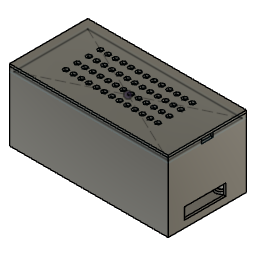
Raspberry Pi Zero W Case v16 (Autodesk Fusion 360 design; units mm, degrees)
Autodesk Fusion 360 part; units mm, degrees
note: some values were not read from the file. Chosen so that the rebuilt part matches the saved one: which face or edge a step refers to.
box "BoxPrimitive1" add length 34 width 69 height 30 placed x (0, -1, 0) y (1, 0, 0) z (0, 0, 1) at (-30, 15, 0) makes body 1
move_body "Align2" bodies 1 to x (1, 0, 0) y (0, 1, 0) z (0, 0, 1) at (-4.5, 2, 0)
shell "Shell1" thickness 1 removed faces 1 at (11.5, 5.6667, 30) on bodies 1
sketch "Sketch2" plane through (0, 0, 1) normal (0, 0, 1) x (-1, 0, 0)
  line L0 (33.5, 16) -> (-33.5, 16)
  line L1 (-33.5, 16) -> (-33.5, -16)
  line L2 (-33.5, -16) -> (33.5, -16)
  line L3 (33.5, -16) -> (33.5, 16)
  circle A0 centre (29, -11.5) radius 2.5
  circle A1 centre (29, -11.5) radius 1.25
  circle A2 through (29.5, -11.5, 4) (28.75, -11.067, 4) (28.75, -11.933, 4)
  dimension "d7" = 5
  dimension "d8" = 4.5
  dimension "d9" = 4.5
  dimension "d10" = 2.5
  dimension "d11" = 1
  constraint concentric A0 A1
  measures "d7" diameter of A0
  measures "d8" distance of L2 A0.centre
  measures "d9" distance of L3 A0.centre
  measures "d10" diameter of A1
sketch "Sketch2 (curves 4 mm off its plane)" plane through (0, 0, 5) normal (0, 0, 1) x (-1, 0, 0)
  circle A0 centre (29, -11.5) radius 0.5
loft "Loft1" add profiles "Sketch2", "Sketch2 (curves 4 mm off its plane)" section 1 contours A1 section 2 bodies 1
extrude "Extrude1" add sketch "Sketch2" along normal blind 1 contours A0 bodies 1
pattern_linear "R-Pattern1" count 2 spacing 58 along (1, 0, 0) count 2 spacing 23 along (0, -1, 0) of 4 faces at (-28.2726, 12.4121, 1.4444) (-29.287, 11.6721, 5) (-31.0694, 11.6863, 2) (-31.4876, 11.7489, 1.6667) on bodies 1
sketch "Sketch3" plane through (0, 17, 0) normal (0, 1, 0) x (-1, 0, 0)
  line L0 (-34.5, 30) -> (-34.5, 0)
  line L1 (-34.5, 0) -> (34.5, 0)
  line L2 (34.5, 0) -> (34.5, 30)
  line L3 (34.5, 30) -> (-34.5, 30)
  line L4 (-13.6, 8) -> (-28.6, 8)
  line L5 (-28.6, 8) -> (-28.6, 3)
  line L6 (-28.6, 3) -> (-13.6, 3)
  line L7 (-13.6, 3) -> (-13.6, 8)
  line L8 (-13.6, 8) -> (-28.6, 3) construction
  line L9 (-28.6, 8) -> (-13.6, 3) construction
  line L10 (2.9, 8) -> (12.9, 8)
  line L11 (12.9, 8) -> (12.9, 3)
  line L12 (12.9, 3) -> (2.9, 3)
  line L13 (2.9, 3) -> (2.9, 8)
  line L14 (2.9, 8) -> (12.9, 3) construction
  line L15 (12.9, 8) -> (2.9, 3) construction
  line L16 (25.5, 3) -> (15.5, 3)
  line L17 (15.5, 3) -> (15.5, 8)
  line L18 (15.5, 8) -> (25.5, 8)
  line L19 (25.5, 8) -> (25.5, 3)
  line L20 (25.5, 3) -> (15.5, 8) construction
  line L21 (15.5, 3) -> (25.5, 8) construction
  point P0 (-21.1, 5.5)
  point P1 (7.9, 5.5)
  point P2 (20.5, 5.5)
  dimension "d18" = 15
  dimension "d19" = 5
  dimension "d20" = 13.4
  dimension "d21" = 5.5
  dimension "d22" = 10
  dimension "d23" = 5
  dimension "d24" = 42.4
  dimension "d25" = 5.5
  dimension "d26" = 10
  dimension "d27" = 5
  dimension "d28" = 5.5
  dimension "d29" = 55
  constraint horizontal L4
  constraint perpendicular L4 L5
  constraint parallel L4 L6
  constraint parallel L5 L7
  constraint coincident L8 P0
  constraint coincident L9 P0
  constraint horizontal L10
  constraint perpendicular L10 L11
  constraint parallel L10 L12
  constraint parallel L11 L13
  constraint coincident L14 P1
  constraint coincident L15 P1
  constraint horizontal L16
  constraint perpendicular L16 L17
  constraint parallel L16 L18
  constraint parallel L17 L19
  constraint coincident L20 P2
  constraint coincident L21 P2
  measures "d18" distance of L5.end L6.end
  measures "d19" distance of L4.end L5.end
  measures "d20" distance of L0 P0
  measures "d21" distance of L1 P0
  measures "d22" distance of L11.end L12.end
  measures "d23" distance of L10.end L11.end
  measures "d24" distance of L0 P1
  measures "d25" distance of L1 P1
  measures "d26" distance of L17.end L18.end
  measures "d27" distance of L16.end L17.end
  measures "d28" distance of L1 P2
  measures "d29" distance of L0 P2
sketch "Sketch4" plane through (34.5, 0, 0) normal (1, 0, 0) x (0, 1, 0)
  line L0 (-17, 30) -> (-17, 0)
  line L1 (-17, 0) -> (17, 0)
  line L2 (17, 0) -> (17, 30)
  line L3 (17, 30) -> (-17, 30)
  line L4 (8.1, 8) -> (-9.9, 8)
  line L5 (-9.9, 8) -> (-9.9, 3)
  line L6 (-9.9, 3) -> (8.1, 3)
  line L7 (8.1, 3) -> (8.1, 8)
  line L8 (8.1, 8) -> (-9.9, 3) construction
  line L9 (-9.9, 8) -> (8.1, 3) construction
  line L10 (17, 30) -> (17, 0)
  point P0 (-0.9, 5.5)
  dimension "d30" = 18
  dimension "d31" = 5
  dimension "d32" = 17.9
  dimension "d33" = 5.5
  constraint horizontal L4
  constraint perpendicular L4 L5
  constraint parallel L4 L6
  constraint parallel L5 L7
  constraint coincident L8 P0
  constraint coincident L9 P0
  measures "d30" distance of L5.end L6.end
  measures "d31" distance of L4.end L5.end
  measures "d32" distance of P0 L10
  measures "d33" distance of L1 P0
extrude "Extrude2" cut sketch "Sketch3" against normal blind 1 contours L4 L5 L6 L7 | L10 L11 L12 L13 | L16 L17 L18 L19 bodies 1
extrude "Extrude3" cut sketch "Sketch4" against normal blind 1 contours L4 L5 L6 L7 bodies 1
sketch "Sketch5" plane through (34.5, 0, 0) normal (1, 0, 0) x (0, 1, 0)
  line L0 (-9.9, 8) -> (8.1, 8)
  line L1 (8.1, 8) -> (8.1, 3)
  line L2 (8.1, 3) -> (-9.9, 3)
  line L3 (-9.9, 3) -> (-9.9, 8)
  line L4 (-17, 30) -> (-17, 0)
  line L5 (-17, 0) -> (17, 0)
  line L6 (17, 0) -> (17, 30)
  line L7 (17, 30) -> (-17, 30)
  line L8 (2.5, 30) -> (-2.5, 30)
  line L9 (-2.5, 30) -> (-2.5, 28)
  line L10 (-2.5, 28) -> (2.5, 28)
  line L11 (2.5, 28) -> (2.5, 30)
  line L12 (2.5, 30) -> (-2.5, 28) construction
  line L13 (-2.5, 30) -> (2.5, 28) construction
  point P0 (0, 29)
  dimension "d38" = 5
  dimension "d39" = 2
  dimension "d40" = 17
  dimension "d41" = 1
  constraint horizontal L8
  constraint perpendicular L8 L9
  constraint parallel L8 L10
  constraint parallel L9 L11
  constraint coincident L12 P0
  constraint coincident L13 P0
  measures "d38" distance of L9.end L10.end
  measures "d39" distance of L8.end L9.end
  measures "d40" distance of L4 P0
  measures "d41" distance of L7 P0
extrude "Extrude4" cut sketch "Sketch5" against normal blind 1 contours L7 L8 L9 L10 L11 bodies 1
sketch "Sketch6" plane through (-34.5, 0, 0) normal (-1, 0, 0) x (0, -1, 0)
  line L0 (-17, 30) -> (-17, 0)
  line L1 (-17, 0) -> (17, 0)
  line L2 (17, 0) -> (17, 30)
  line L3 (17, 30) -> (-17, 30)
  line L4 (2.5, 28) -> (-2.5, 28)
  line L5 (-2.5, 28) -> (-2.5, 30)
  line L6 (-2.5, 30) -> (2.5, 30)
  line L7 (2.5, 30) -> (2.5, 28)
  line L8 (2.5, 28) -> (-2.5, 30) construction
  line L9 (-2.5, 28) -> (2.5, 30) construction
  point P0 (0, 29)
  dimension "d44" = 5
  dimension "d45" = 2
  dimension "d46" = 17
  dimension "d47" = 1
  constraint horizontal L4
  constraint perpendicular L4 L5
  constraint parallel L4 L6
  constraint parallel L5 L7
  constraint coincident L8 P0
  constraint coincident L9 P0
  measures "d44" distance of L5.end L6.end
  measures "d45" distance of L4.end L5.end
  measures "d46" distance of L0 P0
  measures "d47" distance of L3 P0
extrude "Extrude5" cut sketch "Sketch6" against normal blind 1 contours L3 L4 L5 L6 L7 bodies 1
sketch "Sketch7" plane through (-34.5, 0, 0) normal (-1, 0, 0) x (0, -1, 0)
  line L0 (2.5, 30) -> (2.5, 28)
  line L1 (2.5, 28) -> (-2.5, 28)
  line L2 (-2.5, 28) -> (-2.5, 30)
  line L3 (-2.5, 30) -> (-17, 30)
  line L4 (-17, 30) -> (-17, 0)
  line L5 (-17, 0) -> (17, 0)
  line L6 (17, 0) -> (17, 30)
  line L7 (17, 30) -> (2.5, 30)
  circle A0 centre (-8.9262, 21.4902) radius 3.25
  dimension "d50" = 6.5
  measures "d50" diameter of A0
extrude "Extrude6" cut sketch "Sketch7" against normal blind 1 contours A0 bodies 1
box "BoxPrimitive2" add length 34 width 69 height 3 placed x (0, 1, 0) y (-1, 0, 0) z (0, 0, 1) at (91, -28, 0) separate body makes body 2
move_body "Align3" bodies 2 to x (1, 0, 0) y (0, 1, 0) z (0, 0, 1) at (-56.5, 11, -3)
move_body "Move1" bodies 2 to x (1, 0, 0) y (0, 1, 0) z (0, 0, 1) at (0, 0, 31)
sketch "Sketch9" plane through (0, 0, 28) normal (0, 0, -1) x (1, 0, 0)
  line L0 (-34.5, -17) -> (34.5, -17)
  line L1 (34.5, -17) -> (34.5, 17)
  line L2 (34.5, 17) -> (-34.5, 17)
  line L3 (-34.5, 17) -> (-34.5, -17)
  line L4 (33.5, -16) -> (-33.5, -16)
  line L5 (-33.5, -16) -> (-33.5, 16)
  line L6 (-33.5, 16) -> (33.5, 16)
  line L7 (33.5, 16) -> (33.5, -16)
  line L8 (33.5, -16) -> (-33.5, 16) construction
  line L9 (-33.5, -16) -> (33.5, 16) construction
  dimension "d58" = 67
  dimension "d59" = 32
  constraint horizontal L4
  constraint perpendicular L4 L5
  constraint parallel L4 L6
  constraint parallel L5 L7
  constraint coincident L8 origin
  constraint coincident L9 origin
  measures "d58" distance of L5.end L6.end
  measures "d59" distance of L4.end L5.end
extrude "Extrude7" cut sketch "Sketch9" against normal blind 2 bodies 2
sketch "Sketch11" plane through (0, 0, 28) normal (0, 0, -1) x (1, 0, 0)
  line L0 (33.5, -16) -> (33.5, 16)
  line L1 (33.5, 16) -> (-33.5, 16)
  line L2 (-33.5, 16) -> (-33.5, -16)
  line L3 (-33.5, -16) -> (33.5, -16)
  line L4 (32.5, 15) -> (-32.5, 15)
  line L5 (-32.5, 15) -> (-32.5, -15)
  line L6 (-32.5, -15) -> (32.5, -15)
  line L7 (32.5, -15) -> (32.5, 15)
  line L8 (32.5, 15) -> (-32.5, -15) construction
  line L9 (-32.5, 15) -> (32.5, -15) construction
  dimension "d66" = 65
  dimension "d67" = 30
  constraint horizontal L4
  constraint perpendicular L4 L5
  constraint parallel L4 L6
  constraint parallel L5 L7
  constraint coincident L8 origin
  constraint coincident L9 origin
  measures "d66" distance of L5.end L6.end
  measures "d67" distance of L4.end L5.end
extrude "Extrude8" cut sketch "Sketch11" against normal blind 2 contours L4 L5 L6 L7 bodies 2
sketch "Sketch12" plane through (0, 0, 30) normal (0, 0, -1) x (1, 0, 0)
  line L0 (32.5, -15) -> (32.5, 15)
  line L1 (32.5, 15) -> (-32.5, 15)
  line L2 (-32.5, 15) -> (-32.5, -15)
  line L3 (-32.5, -15) -> (32.5, -15)
  circle A0 centre (29, -11.5) radius 2.5
  circle A1 centre (29, -11.5) radius 1.25
  line L4 (33.5, -16) -> (33.5, 16)
  line L5 (-33.5, -16) -> (33.5, -16)
  dimension "d70" = 5
  dimension "d71" = 2.5
  dimension "d72" = 4.5
  dimension "d73" = 4.5
  constraint concentric A0 A1
  measures "d70" diameter of A0
  measures "d71" diameter of A1
  measures "d72" distance of A0.centre L4
  measures "d73" distance of A0.centre L5
extrude "Extrude9" add sketch "Sketch12" along normal blind 27 contours A0 bodies 2
pattern_linear "R-Pattern2" count 2 spacing 57 along (-1, 0, 0) count 2 spacing 23 along (0, -1, 0) of "Extrude9"
sketch "Sketch13" plane through (0, 0, 31) normal (0, 0, 1) x (-1, 0, 0)
  line L0 (-34.5, -17) -> (34.5, -17)
  line L1 (34.5, -17) -> (34.5, 17)
  line L2 (34.5, 17) -> (-34.5, 17)
  line L3 (-34.5, 17) -> (-34.5, -17)
  line L4 (19, -8.5774) -> (20, -9.1547)
  line L5 (20, -9.1547) -> (21, -8.5774)
  line L6 (21, -8.5774) -> (21, -7.4226)
  line L7 (21, -7.4226) -> (20, -6.8453)
  line L8 (20, -6.8453) -> (19, -7.4226)
  line L9 (19, -7.4226) -> (19, -8.5774)
  point P0 (20, -8)
extrude "Extrude10" cut sketch "Sketch13" against normal blind 1 contours L4 L5 L6 L7 L8 L9 bodies 2
pattern_linear "R-Pattern3" count 13 spacing 3.3333 along (1, 0, 0) count 4 spacing 5 along (0, -1, 0) of "Extrude10"
